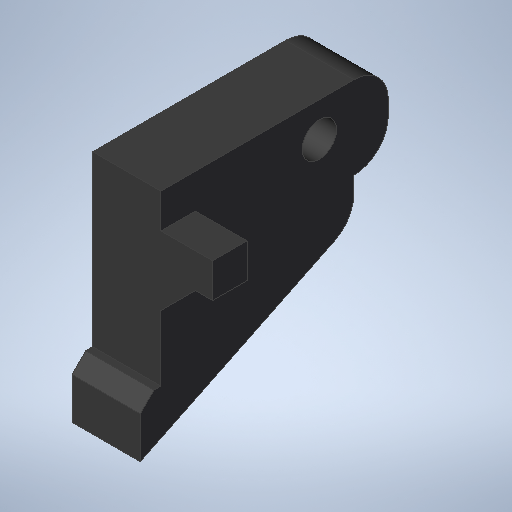
# Autodesk Inventor part: HoldingTri
Saved by Autodesk Inventor 2025 (Build 290162000, 162)
## iProperties
Created: 2025-11-05
Part Number: HoldingTri
Material: Generic
Document SubType Name: Modeling
Designer: ruven
Density: 1 g/cm^3
Appearance: Default
Author: ruven
Autodesk Inventor part; units mm, degrees
ref_plane "YZ Plane" through (0, 0, 0) normal (1, 0, 0) x (0, 1, 0)
ref_plane "XZ Plane" through (0, 0, 0) normal (0, 1, 0) x (-1, 0, 0)
ref_plane "XY Plane" through (0, 0, 0) normal (0, 0, 1) x (1, 0, 0)
sketch "Sketch1" plane through (0, 0, 0) normal (0, 1, 0) x (-1, 0, 0)
  line L0 (-2.45, -18) -> (2.45, -18)
  line L1 (2.45, -18) -> (2.45, 18)
  line L2 (2.45, 18) -> (-2.45, 18)
  line L3 (-2.45, 18) -> (-2.45, -18)
  line L4 (-2.45, -18) -> (2.45, 18) construction
  line L5 (2.45, -18) -> (-2.45, 18) construction
  point P0 (0, 0)
  dimension "d0" = 36
  dimension "d1" = 4.9
  constraints: 12 end point, 2 midpoint, 2 parallel, 1 horizontal, 1 perpendicular
  measures "d0" distance of L0.end L1.end
  measures "d1" distance of L1.end L2.end
extrude "Extrusion1" add sketch "Sketch1" along normal blind 12
sketch "Sketch2" plane through (2.45, 0, 18) normal (1, 0, 0) x (0, 0, -1)
  circle A0 centre (26, 7) radius 2.5
  line L0 (36, 0) -> (36, 12) projected
  line L1 (0, 12) -> (36, 12) projected
  point P0 (18, 0)
  dimension "d4" = 5
  dimension "d5" = 10
  dimension "d18" = 5
  constraints: 1 centre point
  measures "d4" diameter of A0
  measures "d5" distance from line of L0 A0.centre
  measures "d18" distance from line of L1 A0.centre
fillet "Fillet1" radius 5 2 edges at (0, 12, -18) (0, 0, -18)
sketch "Sketch3" plane through (2.45, 0, 18) normal (1, 0, 0) x (0, 0, -1)
  line L0 (0, 0) -> (0, -15)
  arc A0 (36, 7) -> (31, 12) centre (31, 7) ccw projected
  line L1 (0, -15) -> (31, 0)
  line L2 (0, 0) -> (31, 0)
  point P0 (18, 0)
  dimension "d7" = 15
  constraints: 6 end point, 1 horizontal, 1 vertical, 1 other
  measures "d7" distance of L0.start L0.end
extrude "Extrusion2" cut sketch "Sketch2" against normal blind 10
extrude "Extrusion3" add sketch "Sketch3" against normal blind 5
sketch "Skizze4" plane through (2.45, 12, 18) normal (1, 0, 0) x (0, 0, -1)
  line L0 (8, -10) -> (3, -10)
  line L1 (3, -10) -> (3, -5)
  line L2 (3, -5) -> (8, -5)
  line L3 (8, -5) -> (8, -10)
  line L4 (0, 0) -> (31, 0) projected
  line L5 (0, -27) -> (0, 0) projected
  point P0 (18, -12)
  point P1 (3, -7.5)
  dimension "d12" = 5
  dimension "d13" = 5
  dimension "d14" = 5
  dimension "d15" = 3
  constraints: 8 end point, 2 parallel, 1 horizontal, 1 midpoint, 1 perpendicular
  measures "d12" distance of L0.start L0.end
  measures "d13" distance of L0.end L1.end
  measures "d14" distance between parallel lines of L4 L2
  measures "d15" distance from line of point (3, -7.5) L5
extrude "Extrusion4" add sketch "Skizze4" along normal blind 5
sketch "Sketch5" plane through (-2.45, 5, -18) normal (-1, 0, 0) x (0, 0, 1)
  circle A0 centre (10, 2) radius 2.5 projected
  arc A1 (0, 0) -> (5, -5) centre (5, 0) ccw projected
  line L0 (5, -5) -> (36, -5) projected
  line L1 (36, -5) -> (36, 7) projected
  line L2 (5, 7) -> (36, 7) projected
  arc A2 (5, 7) -> (0, 2) centre (5, 2) ccw projected
  line L3 (0, 0) -> (0, 2) projected
  line L4 (5, -5) -> (36, -20) projected
  line L5 (36, -20) -> (36, -5) projected
  line L6 (36, -5) -> (5, -5) projected
  line L7 (5, -5) -> (36, -20) projected
  line L8 (36, -20) -> (36, -5) projected
  line L9 (36, -5) -> (5, -5) projected
  line L10 (5, -5) -> (36, -20) projected
  line L11 (36, -20) -> (36, -5) projected
  line L12 (36, -5) -> (5, -5) projected
  point P0 (18, -5)
extrude "Extrusion5" add sketch "Sketch5" along normal blind 1.5
sketch "Sketch6" plane through (-3.95, 5, -18) normal (-1, 0, 0) x (0, 0, 1)
  line L0 (5, -5) -> (36, -20) projected
  line L1 (36, -20) -> (36, 7) projected
  line L2 (36, 7) -> (5, 7) projected
  arc A0 (5, 7) -> (0, 2) centre (5, 2) ccw projected
  line L3 (0, 2) -> (0, 0) projected
  arc A1 (0, 0) -> (5, -5) centre (5, 0) ccw projected
  circle A2 centre (10, 2) radius 2.5 projected
  point P0 (18, -5)
extrude "Extrusion6" add sketch "Sketch6" along normal blind 0.1
sketch "Sketch7" plane through (2.45, 2, 10) normal (0, -1, 0) x (1, 0, 0)
  line L0 (0, 0) -> (0, 5) projected
  line L1 (0, 0) -> (5, 0) projected
  line L2 (5, 5) -> (5, 0) projected
  line L3 (0, 5) -> (5, 5) projected
  point P0 (-2.45, -10)
extrude "Extrusion7" add sketch "Sketch7" along normal blind 5
chamfer "Chamfer1" distance 5 angle 45 1 edges at (7.45, -3, 12.5)
sketch "Sketch8" plane through (-4.05, 5, -18) normal (-1, 0, 0) x (0, 0, 1)
  line L0 (36, -20) -> (36, 7) projected
  line L1 (36, 7) -> (5, 7) projected
  arc A0 (5, 7) -> (0, 2) centre (5, 2) ccw projected
  line L2 (0, 2) -> (0, 0) projected
  arc A1 (0, 0) -> (5, -5) centre (5, 0) ccw projected
  line L3 (5, -5) -> (36, -20) projected
  circle A2 centre (10, 2) radius 2.5 projected
  point P0 (18, -5)
extrude "Extrusion8" add sketch "Sketch8" along normal blind 3.4
sketch "Sketch9" plane through (7.45, 12, 18) normal (1, 0, 0) x (0, 0, -1)
  line L0 (8, -10) -> (3, -10) construction
  line L1 (8, -5) -> (8, -10) construction
  line L2 (8, -5) -> (3, -5) construction
  line L3 (3, -5) -> (3, -10) construction
  line L4 (8, -10) -> (3, -10) projected
  line L5 (8, -5) -> (8, -10) projected
  line L6 (8, -5) -> (3, -5) projected
  line L7 (3, -5) -> (3, -10) projected
  point P0 (18, -12)
extrude "Extrusion9" add sketch "Sketch9" along normal blind 2.5
sketch "Sketch10" plane through (-7.45, 0, -13) normal (0, -0.9001593, -0.4355609) x (1, 0, 0)
  point P0 (7.45, 11.7021)
sketch "Sketch11" plane through (-7.45, 0, -13) normal (0, -0.9001593, -0.4355609) x (1, 0, 0)
  point P0 (7.45, 11.7021)
sketch "Sketch12" plane through (-7.45, 5, -18) normal (-1, 0, 0) x (0, 0, 1)
  line L0 (36, -20) -> (36, -25.5)
  line L1 (36, -25.5) -> (5, -10.5)
  line L2 (5, -10.5) -> (5, -5)
  arc A0 (0, 0) -> (5, -5) centre (5, 0) ccw projected
  line L3 (5, -5) -> (36, -20)
  point P0 (18, -5)
  dimension "d32" = 5.5
  dimension "d33" = 5.5
  constraints: 8 end point, 1 parallel, 1 vertical
  measures "d32" distance of L1.end L2.end
  measures "d33" distance of L0.start L0.end
extrude "Extrusion10" add sketch "Sketch12" against normal blind 9.9
fillet "Fillet2" radius 5 1 edges at (-2.5, -5.5, -13)
fillet "Fillet3" [suppressed]
sketch "Sketch13" plane through (2.45, 5, -18) normal (1, 0, 0) x (0, 0, -1)
  line L0 (-36, 7) -> (-36, -25.5) projected
  line L1 (-36, 7) -> (-33, 7)
  line L2 (-33, 7) -> (-33, -17.5)
  line L3 (-33, -17.5) -> (-36, -17.5)
  line L4 (-36, -17.5) -> (-36, 7)
  point P0 (-18, -5)
  point P1 (-36, -17.5)
  dimension "d40" = 24.5
  constraints: 8 end point, 2 parallel, 1 horizontal, 1 perpendicular
  measures "d40" distance between parallel lines of L3 L1
extrude "Extrusion11" cut sketch "Sketch13" against normal blind 10
chamfer "Chamfer2" distance 2 angle 45 1 edges at (-5.75, -12.5, 18)
body "Solid1"
